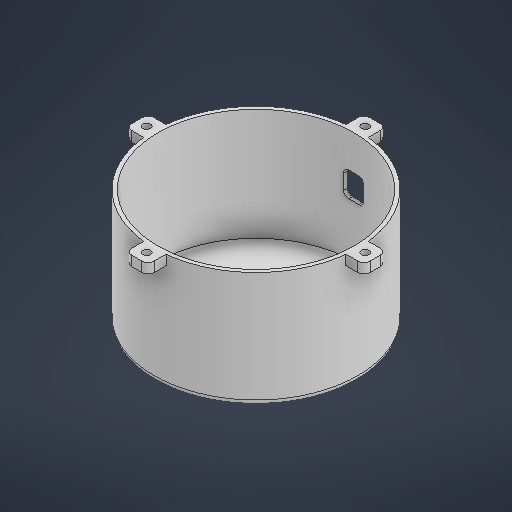
# Autodesk Inventor part: ruka base
Saved by Autodesk Inventor 2026 (Build 300175000, 175)
## iProperties
Created: 2025-04-11
Part Number: ruka base
Material: Generic
Document SubType Name: Modeling
Designer: janpa
Density: 1 g/cm^3
Appearance: Default
Author: janpa
Autodesk Inventor part; units mm, degrees
ref_plane "YZ Plane" through (0, 0, 0) normal (1, 0, 0) x (0, 1, 0)
ref_plane "XZ Plane" through (0, 0, 0) normal (0, 1, 0) x (-1, 0, 0)
ref_plane "XY Plane" through (0, 0, 0) normal (0, 0, 1) x (1, 0, 0)
sketch "Sketch1" plane through (0, 0, 0) normal (0, 1, 0) x (-1, 0, 0)
  circle A0 centre (0, 0) radius 41
  dimension "d0" = 82
  constraints: 1 centre point, 1 coincident
  measures "d0" diameter of A0
extrude "Extrusion1" add sketch "Sketch1" along normal blind 1.5
sketch "Sketch2" plane through (0, 1.5, 0) normal (0, 1, 0) x (1, 0, 0)
  circle A0 centre (0, 0) radius 41
  circle A1 centre (0, 0) radius 39.5
  circle A2 centre (0, 0) radius 6.7
  circle A3 centre (0, 0) radius 2.5
  dimension "d3" = 82
  dimension "d4" = 79
  dimension "d5" = 13.4
  dimension "d6" = 5
  constraints: 4 centre point, 4 coincident
  measures "d3" diameter of A0
  measures "d4" diameter of A1
  measures "d5" diameter of A2
  measures "d6" diameter of A3
extrude "Extrusion2" add sketch "Sketch2" along normal blind 45 contours A0
extrude "Extrusion3" cut sketch "Sketch2" along normal mid plane 45 contours A2 | A3
fillet "Fillet1" radius 2 1 edges at (41, 0, 0)
sketch "Sketch3" plane through (0, 46.5, 0) normal (0, 1, 0) x (1, 0, 0)
  line L0 (-40, -4.5) -> (-45.5, -4.5)
  line L1 (-48, -2) -> (-48, 2)
  line L2 (-45.5, 4.5) -> (-40, 4.5)
  line L3 (-40, 4.5) -> (-40, -4.5)
  circle A0 centre (-44, 0) radius 1.5
  circle A1 centre (-44, 0) radius 2.8
  arc A2 (-48, -2) -> (-45.5, -4.5) centre (-45.5, -2) ccw
  arc A3 (-45.5, 4.5) -> (-48, 2) centre (-45.5, 2) ccw
  line L4 (-57.15, -71.4375) -> (-33.3375, -71.4375)
  line L5 (-33.3375, -71.4375) -> (-33.3375, -57.15)
  line L6 (-4.5, -40) -> (4.5, -40)
  line L7 (4.5, -40) -> (4.5, -45.5)
  line L8 (-4.5, -45.5) -> (-4.5, -40)
  circle A4 centre (0, -44) radius 1.5
  circle A5 centre (0, -44) radius 2.8
  line L9 (2, -48) -> (-2, -48)
  arc A6 (-4.5, -45.5) -> (-2, -48) centre (-2, -45.5) ccw
  arc A7 (2, -48) -> (4.5, -45.5) centre (2, -45.5) ccw
  line L10 (40, -4.5) -> (40, 4.5)
  line L11 (40, 4.5) -> (45.5, 4.5)
  line L12 (45.5, -4.5) -> (40, -4.5)
  circle A8 centre (44, 0) radius 1.5
  circle A9 centre (44, 0) radius 2.8
  line L13 (48, 2) -> (48, -2)
  arc A10 (45.5, -4.5) -> (48, -2) centre (45.5, -2) ccw
  arc A11 (48, 2) -> (45.5, 4.5) centre (45.5, 2) ccw
  line L14 (4.5, 40) -> (-4.5, 40)
  line L15 (-4.5, 40) -> (-4.5, 45.5)
  line L16 (4.5, 45.5) -> (4.5, 40)
  circle A12 centre (0, 44) radius 1.5
  circle A13 centre (0, 44) radius 2.8
  line L17 (-2, 48) -> (2, 48)
  arc A14 (4.5, 45.5) -> (2, 48) centre (2, 45.5) ccw
  arc A15 (-2, 48) -> (-4.5, 45.5) centre (-2, 45.5) ccw
  point P0 (0, 0)
  point P1 (-48, 4.5)
  point P2 (-48, -4.5)
  point P3 (4.5, -48)
  point P4 (-4.5, -48)
  point P5 (48, 4.5)
  point P6 (48, -4.5)
  point P7 (-4.5, 48)
  point P8 (4.5, 48)
  dimension "d12" = 8
  dimension "d13" = 9
  dimension "d14" = 4.5
  dimension "d15" = 40
  dimension "d16" = 3
  dimension "d17" = 5.6
  dimension "d18" = 2.5
  dimension "d19" = 4
  dimension "d22" = 360
  constraints: 36 end point, 16 centre point, 16 point on circle, 16 point on line, 4 coincident, 4 tangent, 2 horizontal, 2 parallel, 2 perpendicular, 1 equal radius, 81 other
  measures "d12" distance of point (-48, 4.5) L2.end
  measures "d13" distance of point (-48, -4.5) point (-48, 4.5)
  measures "d14" distance from line of point (0, 0) L2
  measures "d15" distance from line of point (0, 0) L3
  measures "d16" diameter of A0
  measures "d17" diameter of A1
  measures "d18" radius of A2
  measures "d19" distance from line of L3 A1.centre
extrude "Extrusion4" add sketch "Sketch3" against normal blind 4 contours L0 A2 L1 A3 L2 L3 | A1 | L6 L7 A7 L9 A6 L8 | A5 | L10 L11 A11 L13 A10 L12 | A9 | L14 L15 A15 L17 A14 L16 | A13
sketch "Sketch4" plane through (0, 42.5, 0) normal (0, -1, 0) x (1, 0, 0)
  circle A0 centre (0, 44) radius 1.5 projected
  circle A1 centre (0, 44) radius 2.75
  circle A2 centre (-44, 0) radius 2.75
  circle A3 centre (0, -44) radius 2.75
  circle A4 centre (44, 0) radius 2.75
  point P0 (0, 0)
  dimension "d26" = 5.5
  dimension "d29" = 360
  constraints: 4 centre point, 1 coincident, 9 other
  measures "d26" diameter of A1
extrude "Extrusion5" cut sketch "Sketch4" against normal blind 1
sketch "Sketch5" plane through (0, 0, 0) normal (0, -1, 0) x (1, 0, 0)
  circle A0 centre (-4.75, 35.61) radius 1.5
  line L0 (41.275, 69.85) -> (41.275, 62.6049)
  line L1 (41.275, 62.6049) -> (35.5703, 62.6049)
  circle A1 centre (4.75, 35.61) radius 1.5
  circle A2 centre (-4.75, -14.39) radius 1.5
  circle A3 centre (4.75, -14.39) radius 1.5
  line L2 (48, -2) -> (48, 2) projected
  point P0 (0, 0)
  dimension "d33" = 3
  dimension "d36" = 9.5
  dimension "d39" = 50
  dimension "d42" = 52.75
  dimension "d43" = -14.39
  constraints: 4 centre point, 4 end point, 2 vertical, 1 horizontal, 1 perpendicular
  measures "d33" diameter of A0
  measures "d36" distance of A0.centre A1.centre
  measures "d39" distance of A0.centre A2.centre
  measures "d42" distance from line of L2 A0.centre
  measures "d43" vertical distance of point (0, 0) A2.centre
extrude "Extrusion6" cut sketch "Sketch5" against normal blind 20
sketch "Sketch6" plane through (0, 0, 0) normal (0, -1, 0) x (1, 0, 0)
  circle A0 centre (-4.75, 35.61) radius 1.5 projected
  circle A1 centre (-4.75, 35.61) radius 2.8
  line L0 (-57.15, 46.0375) -> (-53.975, 46.0375)
  line L1 (-53.975, 46.0375) -> (-53.975, 48.8108)
  circle A2 centre (4.75, 35.61) radius 2.8
  circle A3 centre (-4.75, -14.39) radius 2.8
  circle A4 centre (4.75, -14.39) radius 2.8
  point P0 (0, 0)
  dimension "d46" = 5.6
  dimension "d49" = 9.5
  dimension "d52" = 50
  constraints: 4 centre point, 4 end point, 1 coincident, 1 horizontal, 1 perpendicular, 1 vertical, 6 other
  measures "d46" diameter of A1
  measures "d49" distance of A1.centre A2.centre
  measures "d52" distance of A1.centre A3.centre
extrude "Extrusion7" cut sketch "Sketch6" against normal blind 1 contours A0 | A1 | A2 | A3 | A4
sketch "Sketch7" plane through (2, 46.5, -48) normal (0, 0, -1) x (-1, 0, 0)
  line L0 (6, -24) -> (-2, -24)
  line L1 (-2, -24) -> (-2, -14)
  line L2 (-2, -14) -> (6, -14)
  line L3 (6, -14) -> (6, -24)
  line L4 (4, -4) -> (0, -4) projected
  line L5 (6.5, 0) -> (6.5, -4) projected
  line L6 (-2.5, 0) -> (-2.5, -4) projected
  point P0 (2, -46.5)
  point P1 (2, -14)
  dimension "d57" = 10
  dimension "d58" = 10
  dimension "d59" = 8
  dimension "d64" = 0.5
  constraints: 8 end point, 2 parallel, 1 horizontal, 1 midpoint, 1 perpendicular
  measures "d57" distance from line of L4 point (2, -14)
  measures "d58" distance of L2.end L0.start
  measures "d59" distance of L0.start L0.end
  measures "d64" distance between parallel lines of L5 L3
extrude "Extrusion8" cut sketch "Sketch7" against normal blind 50
fillet "Fillet2" radius 2 4 edges at (4, 22.5, -40.0507) (-4, 22.5, -40.0507) (4, 32.5, -40.0507) (-4, 32.5, -40.0507)
body "Solid1"
